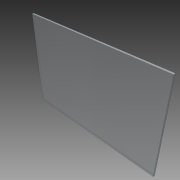
# Autodesk Inventor part: main_lcd_cover_glass
Saved by Autodesk Inventor 2014 (Build 180170000, 170)
## iProperties
Created: 2014-03-22
Part Number: main_lcd_cover_glass
Material: Glass
Document SubType Name: Modeling
Designer: buben
Density: 2.18 g/cm^3
Appearance: Clear
Author: buben
Autodesk Inventor part; units mm, degrees
ref_plane "YZ Plane" through (0, 0, 0) normal (1, 0, 0) x (0, 1, 0)
ref_plane "XZ Plane" through (0, 0, 0) normal (0, 1, 0) x (-1, 0, 0)
ref_plane "XY Plane" through (0, 0, 0) normal (0, 0, 1) x (1, 0, 0)
sketch "Sketch1" plane through (0, 0, 0) normal (0, 1, 0) x (-1, 0, 0)
  line L0 (0, 0) -> (-162, 0)
  line L1 (-162, 0) -> (-162, -108)
  line L2 (-162, -108) -> (0, -108)
  line L3 (0, -108) -> (0, 0)
  dimension "d0" = 162
  dimension "d1" = 108
  constraints: 8 end point, 2 parallel, 1 horizontal, 1 perpendicular
  measures "d0" distance of L0.start L0.end
  measures "d1" distance of L2.end L0.start
extrude "Extrusion1" add sketch "Sketch1" along normal blind 2
chamfer "Chamfer1" distance 0.3 angle 45 12 edges at (81, 2, 0) (0, 2, -54) (162, 2, -54) (81, 2, -108) (162, 0, -54) (81, 0, 0) (0, 0, -54) (81, 0, -108) (0, 1, 0) (0, 1, -108) (162, 1, 0) (162, 1, -108)
body "Solid1"
